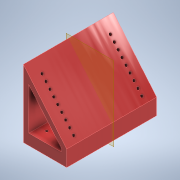
# Autodesk Inventor part: bracketForGarageMiddlePiece
Saved by Autodesk Inventor 2022.1 (Build 261234020, 234B)
## iProperties
Created: 2021-10-20
Part Number: bracketForGarageMiddlePiece
Material: PC/ABS Plastic
Document SubType Name: Modeling
Designer: robst
Density: 0.357273 g/cm^3
Appearance: Red
Author: robst
Autodesk Inventor part; units mm, degrees
ref_plane "YZ Plane" through (0, 0, 0) normal (1, 0, 0) x (0, 1, 0)
ref_plane "XZ Plane" through (0, 0, 0) normal (0, 1, 0) x (-1, 0, 0)
sketch "Sketch49" plane through (0, 0, 0) normal (0, 0, 1) x (1, 0, 0)
  line L0 (0, 0) -> (0, 150) construction
  line L1 (0, 0) -> (40, 0)
  line L2 (40, 0) -> (40, 29.6597)
  line L3 (40, 29.6597) -> (-40, 125)
  line L4 (-40, 125) -> (-40, 0)
  line L5 (-40, 0) -> (0, 0)
  dimension "d222" = 40
  dimension "d223" = 40
  dimension "d225" = 125
  constraints: 12 end point, 2 perpendicular, 1 collinear, 1 horizontal, 1 parallel, 1 point on line, 1 vertical
  measures "d222" distance between parallel lines of L2 L0
  measures "d223" angle of L3 L4
  measures "d225" distance of L3.end L4.end
extrude "Extrusion22" add sketch "Sketch49" along normal mid plane 166
sketch "Sketch50" plane through (-40, 0, 83) normal (0, -1, 0) x (1, 0, 0)
  line L0 (23, -146) -> (57, -146) construction
  line L1 (57, -146) -> (57, -20) construction
  line L2 (57, -20) -> (23, -20) construction
  line L3 (23, -20) -> (23, -146) construction
  line L4 (23, -146) -> (57, -20) construction
  line L5 (57, -146) -> (23, -20) construction
  point P0 (40, -83)
  point P1 (23, -146)
  point P2 (57, -146)
  dimension "d228" = 126
  dimension "d229" = 34
  dimension "d248" = 126
  dimension "d251" = 34
  constraints: 12 end point, 2 horizontal, 2 midpoint, 2 parallel, 1 coincident, 1 perpendicular, 1 vertical, 3 other
  measures "d228" distance of L2.end L0.start
  measures "d229" distance of L1.end L2.end
  measures "d248" distance of point (23, -20) point (23, -146)
  measures "d251" distance of point (23, -20) point (57, -20)
sketch "Sketch52" plane through (-40, 125, 83) normal (0.7660444, 0.6427876, 0) x (0, 0, -1)
  line L0 (166, 0) -> (0, 0) projected
  line L1 (0, -124.4579) -> (0, 0) projected
  line L2 (166, -124.4579) -> (0, -124.4579) projected
  line L3 (166, 0) -> (166, -124.4579) projected
  line L4 (0, -23) -> (166, -23) construction
  line L5 (20, 0) -> (20, -124.4579) construction
  point P0 (83, -121.4671)
  point P1 (20, -23)
  point P2 (146, -23)
  point P3 (20, -34.3333)
  point P4 (146, -34.3333)
  point P5 (20, -45.6667)
  point P6 (146, -45.6667)
  point P7 (20, -57)
  point P8 (146, -57)
  point P9 (20, -68.3333)
  point P10 (146, -68.3333)
  point P11 (20, -79.6667)
  point P12 (146, -79.6667)
  point P13 (20, -91)
  point P14 (146, -91)
  point P15 (20, -102.3333)
  point P16 (146, -102.3333)
  point P17 (20, -113.6667)
  point P18 (146, -113.6667)
  dimension "d230" = 20
  dimension "d231" = 23
  dimension "d234" = 126
  dimension "d237" = 11.3333
  constraints: 6 point on line, 4 end point, 2 perpendicular, 1 horizontal, 1 vertical, 17 other
  measures "d230" distance between parallel lines of L5 L1
  measures "d231" distance between parallel lines of L4 L0
  measures "d234" distance of point (20, -23) point (146, -23)
  measures "d237" distance of point (20, -23) point (20, -34.333)
sketch "Sketch53" plane through (0, 0, 83) normal (0, 0, 1) x (1, 0, 0)
  line L0 (40, 29.6597) -> (-40, 125) projected
  line L1 (40, 0) -> (40, 29.6597) projected
  line L2 (-40, 0) -> (40, 0) projected
  line L3 (-40, 125) -> (-40, 0) projected
  line L4 (-30, 20) -> (30, 20)
  line L5 (30, 20) -> (30, 26.02)
  line L6 (30, 26.02) -> (-30, 97.5252)
  line L7 (-30, 97.5252) -> (-30, 20)
  point P0 (0, 0)
  point P1 (30, 23.01)
  dimension "d240" = 20
  dimension "d241" = 10
  dimension "d242" = 10
  dimension "d243" = 10
  constraints: 8 end point, 2 parallel, 1 horizontal, 1 midpoint, 1 perpendicular
  measures "d240" distance between parallel lines of L4 L2
  measures "d241" distance between parallel lines of L7 L3
  measures "d242" distance between parallel lines of L6 L0
  measures "d243" distance from line of point (30, 23.01) L1
extrude "Extrusion23" cut sketch "Sketch53" against normal blind 40 contours L7 L6 L5 L4
mirror "Mirror3" about plane through (0, 0, 0) normal (0, 0, 1) of "Extrusion23"
hole "Hole6" at (-17, 0, 63) at (-17, 0, -63) at (17, 0, 63) at (17, 0, -63) direction (0, 1, 0) diameter 5.105 depth 20 tip angle 118 clearance for "Flat Head Machine Screw (82)" size "#10" standard "Ansi Unified Screw Threads"
hole "Hole7" at (-25.2159, 107.381, 63) at (-25.2159, 107.381, -63) at (-17.931, 98.6991, 63) at (-17.931, 98.6991, -63) at (-10.646, 90.0173, 63) at (-10.646, 90.0173, -63) at (-3.3611, 81.3355, 63) at (-3.3611, 81.3355, -63) at (3.9238, 72.6536, 63) at (3.9238, 72.6536, -63) at (11.2087, 63.9718, 63) at (11.2087, 63.9718, -63) at (18.4937, 55.29, 63) at (18.4937, 55.29, -63) at (25.7786, 46.6081, 63) at (25.7786, 46.6081, -63) at (33.0635, 37.9263, 63) at (33.0635, 37.9263, -63) direction (-0.7660444, -0.6427876, 0) diameter 5.105 depth 10 clearance for "Flat Head Machine Screw (82)" size "#10" standard "Ansi Unified Screw Threads"
equation "\"wallThickness\" = 8"
equation "\"twoByFourWidth\" = 40.64"
equation "\"twoByFourDepth\" = 84.1375"
equation "\"azimuth\" = -15deg"
equation "\"elevation\" = 20deg"
equation "\"depthOfExtrusionForMatingToLowerHalf\" = 12.5"
equation "\"depthForWasherForMatingToCase\" = 14"
body "Solid3"
